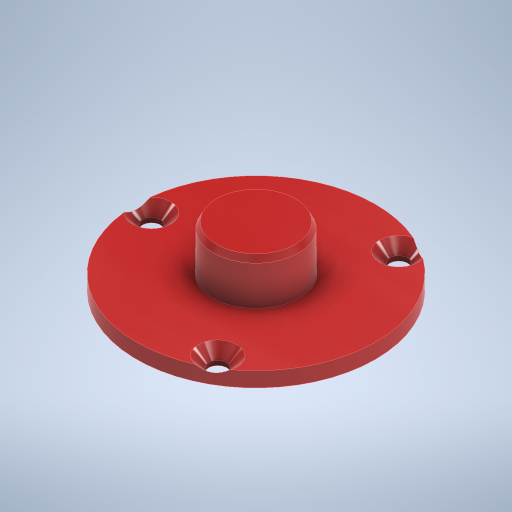
# Autodesk Inventor part: WindFoot
Saved by Autodesk Inventor 2024.3 (Build 283343000, 343)
## iProperties
Created: 2024-11-20
Part Number: WindFoot
Material: PET-Kunststoff
Document SubType Name: Modeling
Designer: Maximilian Hock
Density: 1.541 g/cm^3
Appearance: Rot
Author: Maximilian Hock
## iProperties of the stored document WindFoot_3D-Druck.ipt
Created: 2024-12-16
Part Number: WindFoot_3D-Druck
Material: Generisch
Document SubType Name: Modeling
Designer: Maximilian Hock
Density: 1 g/cm^3
Appearance: Vorgabe
Author: Maximilian Hock
Autodesk Inventor part; units mm, degrees
ref_plane "YZ Plane" through (0, 0, 0) normal (1, 0, 0) x (0, 1, 0)
ref_plane "XZ Plane" through (0, 0, 0) normal (0, 1, 0) x (-1, 0, 0)
ref_plane "XY Plane" through (0, 0, 0) normal (0, 0, 1) x (1, 0, 0)
sketch "Skizze1" plane through (0, 0, 0) normal (0, 0, 1) x (1, 0, 0)
  circle A0 centre (0, 0) radius 40
  dimension "d0" = 80
  constraints: 1 centre point, 1 coincident
  measures "d0" diameter of A0
extrude "Extrusion1" add sketch "Skizze1" along normal blind 5
sketch "Skizze2" plane through (0, 0, 5) normal (0, 0, 1) x (1, 0, 0)
  circle A0 centre (0, 0) radius 14.5
  dimension "d3" = 29
  constraints: 1 centre point, 1 coincident
  measures "d3" diameter of A0
extrude "Extrusion2" add sketch "Skizze2" along normal blind 15 draft -1
sketch "Skizze3" plane through (0, 0, 5) normal (0, 0, 1) x (1, 0, 0)
  circle A0 centre (0, 0) radius 35 construction
  line L0 (-35, 0) -> (17.5, -30.3109) construction
  line L1 (17.5, 30.3109) -> (17.5, -30.3109) construction
  line L2 (17.5, 30.3109) -> (-35, 0) construction
  dimension "d6" = 70
  constraints: 6 end point, 3 point on circle, 2 equal length, 1 centre point, 1 coincident, 1 horizontal alignment
  measures "d6" diameter of A0
hole "Bohrung1" at (-35, 0, 5) at (17.5, 30.3109, 5) at (17.5, -30.3109, 5) direction (0, 0, -1) diameter 6.1 end through all countersink diameter 13 countersink angle 90
chamfer "Fasen1" distance 1 distance2 2 1 edges at (-14.2382, 0, 20) measured on face at (3.1468, 0.1942, 20)
sketch "Skizze4" plane through (0, 0, 0) normal (0, 0, -1) x (-1, 0, 0)
  line L0 (0, 0) -> (28.2843, 0) construction
  line L1 (28.2843, 0) -> (28.2843, -28.2843) construction
  line L2 (28.2843, -28.2843) -> (0, -28.2843) construction
  line L3 (0, -28.2843) -> (0, 0) construction
  circle A0 centre (0, 0) radius 40 projected
  line L4 (2.9271, -3.5681) -> (0.3545, -3.5681)
  line L5 (0.3545, -3.5681) -> (0.3545, -2.998)
  spline S0 degree 2 poles (0.3545, -2.998) (0.6807, -2.737) (1.2026, -2.2776) (1.3983, -2.0705) knots 0 0 0 1 2 2 2
  spline S1 degree 2 poles (1.3983, -2.0705) (1.6564, -1.8011) (1.8861, -1.3898) (1.8861, -1.1742) knots 0 0 0 1 2 2 2
  spline S2 degree 2 poles (1.8861, -1.1742) (1.8861, -0.9303) (1.594, -0.6694) (1.3331, -0.6694) knots 0 0 0 1 2 2 2
  spline S3 degree 2 poles (1.3331, -0.6694) (1.1998, -0.6694) (0.9615, -0.7346) (0.8395, -0.7857) knots 0 0 0 1 2 2 2
  spline S4 degree 2 poles (0.8395, -0.7857) (0.7204, -0.8395) (0.5502, -0.953) (0.5077, -0.9814) knots 0 0 0 1 2 2 2
  line L6 (0.5077, -0.9814) -> (0.4396, -0.9814)
  line L7 (0.4396, -0.9814) -> (0.4396, -0.2184)
  spline S5 degree 2 poles (0.4396, -0.2184) (0.5871, -0.1475) (1.2168, 0) (1.5089, 0) knots 0 0 0 1 2 2 2
  spline S6 degree 2 poles (1.5089, 0) (2.1329, 0) (2.7739, -0.5559) (2.7739, -1.0579) knots 0 0 0 1 2 2 2
  spline S7 degree 2 poles (2.7739, -1.0579) (2.7739, -1.3671) (2.4818, -1.9627) (2.1442, -2.3031) knots 0 0 0 1 2 2 2
  spline S8 degree 2 poles (2.1442, -2.3031) (1.9315, -2.513) (1.5316, -2.8391) (1.4437, -2.9072) knots 0 0 0 1 2 2 2
  line L8 (1.4437, -2.9072) -> (2.9271, -2.9072)
  line L9 (2.9271, -2.9072) -> (2.9271, -3.5681)
  line L10 (4.2318, -3.5681) -> (3.4007, -3.5681)
  line L11 (3.4007, -3.5681) -> (3.4007, -2.6434)
  line L12 (3.4007, -2.6434) -> (4.2318, -2.6434)
  line L13 (4.2318, -2.6434) -> (4.2318, -3.5681)
  line L14 (7.3404, -3.5681) -> (5.0288, -3.5681)
  line L15 (5.0288, -3.5681) -> (5.0288, -2.9583)
  line L16 (5.0288, -2.9583) -> (5.7662, -2.9583)
  line L17 (5.7662, -2.9583) -> (5.7662, -1.1062)
  line L18 (5.7662, -1.1062) -> (5.0288, -1.1062)
  line L19 (5.0288, -1.1062) -> (5.0288, -0.5361)
  spline S9 degree 2 poles (5.0288, -0.5361) (5.1904, -0.5361) (5.5109, -0.4935) (5.6074, -0.4481) knots 0 0 0 1 2 2 2
  spline S10 degree 2 poles (5.6074, -0.4481) (5.718, -0.3914) (5.8428, -0.2014) (5.8541, -0.0596) knots 0 0 0 1 2 2 2
  line L20 (5.8541, -0.0596) -> (6.6199, -0.0596)
  line L21 (6.6199, -0.0596) -> (6.6199, -2.9583)
  line L22 (6.6199, -2.9583) -> (7.3404, -2.9583)
  line L23 (7.3404, -2.9583) -> (7.3404, -3.5681)
  line L24 (8.8011, -3.5681) -> (7.97, -3.5681)
  line L25 (7.97, -3.5681) -> (7.97, -2.6434)
  line L26 (7.97, -2.6434) -> (8.8011, -2.6434)
  line L27 (8.8011, -2.6434) -> (8.8011, -3.5681)
  line L28 (11.9096, -3.5681) -> (9.5981, -3.5681)
  line L29 (9.5981, -3.5681) -> (9.5981, -2.9583)
  line L30 (9.5981, -2.9583) -> (10.3355, -2.9583)
  line L31 (10.3355, -2.9583) -> (10.3355, -1.1062)
  line L32 (10.3355, -1.1062) -> (9.5981, -1.1062)
  line L33 (9.5981, -1.1062) -> (9.5981, -0.5361)
  spline S11 degree 2 poles (9.5981, -0.5361) (9.7597, -0.5361) (10.0802, -0.4935) (10.1767, -0.4481) knots 0 0 0 1 2 2 2
  spline S12 degree 2 poles (10.1767, -0.4481) (10.2873, -0.3914) (10.4121, -0.2014) (10.4234, -0.0596) knots 0 0 0 1 2 2 2
  line L34 (10.4234, -0.0596) -> (11.1892, -0.0596)
  line L35 (11.1892, -0.0596) -> (11.1892, -2.9583)
  line L36 (11.1892, -2.9583) -> (11.9096, -2.9583)
  line L37 (11.9096, -2.9583) -> (11.9096, -3.5681)
  constraints: 1 coincident, 1 horizontal, 1 perpendicular, 4 other
emboss "Prägen1" sketch "Skizze4" operation cut depth 0.5 direction (0, 0, 1) contours L4 L5 S0 S1 S2 S3 S4 L6 L7 S5 S6 S7 S8 L8 L9 | L10 L11 L12 L13 | L14 L15 L16 L17 L18 L19 S9 S10 L20 L21 L22 L23 | L24 L25 L26 L27 | L28 L29 L30 L31 L32 L33 S11 S12 L34 L35 L36 L37
equation "\"d0\" = WindFootDiameter"
equation "\"d1\" = WindFootThickness"
equation "\"d3\" = WindTowerInnerDiameter"
equation "\"WindFootDiameter\" = 80"
equation "\"WindFootThickness\" = 5"
equation "\"WindTowerInnerDiameter\" = 29"
